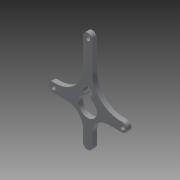
# Autodesk Inventor part: Fish Rib
Saved by Autodesk Inventor 2015 (Build 190159000, 159)
## iProperties
Created: 2014-11-02
Part Number: Fish Rib
Material: Generic
Document SubType Name: Modeling
Designer: Ryan
Density: 1 g/cm^3
Appearance: Default
Mass: 1.22571 g
Surface Area: 15.6256 cm^2
Volume: 1.22571 cm^3
Author: Ryan
Autodesk Inventor part; units mm, degrees
ref_plane "YZ Plane" through (0, 0, 0) normal (1, 0, 0) x (0, 1, 0)
ref_plane "XZ Plane" through (0, 0, 0) normal (0, 1, 0) x (-1, 0, 0)
ref_plane "XY Plane" through (0, 0, 0) normal (0, 0, 1) x (1, 0, 0)
sketch "Sketch1" plane through (0, 0, 0) normal (0, 0, 1) x (1, 0, 0)
  line L0 (0, 0) -> (0, 25.4)
  line L1 (0, 0) -> (0, -25.4)
  line L2 (-19.0266, -7.6091) -> (19.0734, -7.6091)
  circle A0 centre (0, 0) radius 2.54
  circle A1 centre (0, 25.4) radius 2.54
  circle A2 centre (-19.0266, -7.6091) radius 2.54
  circle A3 centre (19.0734, -7.6091) radius 2.54
  circle A4 centre (0, -25.4) radius 2.54
  circle A5 centre (0.0234, -7.6091) radius 5.08
  arc A6 (-1.9812, -2.9413) -> (-1.7729, -1.8189) centre (-2.2521, -2.3105) ccw
  arc A7 (1.7485, -1.8423) -> (1.9483, -2.9079) centre (2.1929, -2.3105) ccw
  line L3 (-2.54, 25.4) -> (-2.54, 10.1709)
  line L4 (2.54, 25.4) -> (2.54, 10.1709)
  line L5 (-2.54, -25.4) -> (-2.54, -19.0391)
  line L6 (2.54, -25.4) -> (2.54, -19.0391)
  line L7 (19.0734, -10.1491) -> (11.43, -10.1491)
  line L8 (19.0734, -5.0691) -> (17.78, -5.0691)
  line L9 (-19.0266, -5.0691) -> (-17.78, -5.0691)
  line L10 (-19.0266, -10.1491) -> (-11.43, -10.1491)
  arc A8 (-17.78, -5.0691) -> (-2.54, 10.1709) centre (-17.78, 10.1709) ccw
  arc A9 (2.54, 10.1709) -> (17.78, -5.0691) centre (17.78, 10.1709) ccw
  arc A10 (-2.54, -19.0391) -> (-11.43, -10.1491) centre (-11.43, -19.0391) ccw
  arc A11 (11.43, -10.1491) -> (2.54, -19.0391) centre (11.43, -19.0391) ccw
  circle A12 centre (-19.0266, -7.6091) radius 1.27
  circle A13 centre (0, 25.4) radius 1.27
  circle A14 centre (19.0734, -7.6091) radius 1.27
  dimension "d0" = 25.4
  dimension "d1" = 25.4
  dimension "d2" = 38.1
  dimension "d3" = 38.1
  dimension "d5" = 5.08
  dimension "d6" = 5.08
  dimension "d7" = 5.08
  dimension "d8" = 5.08
  dimension "d9" = 7.6091
  dimension "d10" = 5.08
  dimension "d12" = 4.445
  dimension "d13" = 35.56
  dimension "d14" = 22.86
  dimension "d15" = 10.16
  dimension "d16" = 2.54
  dimension "d17" = 2.54
  dimension "d18" = 2.54
  constraints: 24 point on circle, 23 end point, 20 tangent, 15 centre point, 8 coincident, 6 vertical, 5 horizontal, 3 horizontal alignment, 1 midpoint
  measures "d0" distance of L0.end L0.start
  measures "d1" distance of L0.start L1.end
  measures "d2" distance of L0.end L2.start
  measures "d3" distance of L2.start L2.end
  measures "d5" diameter of A4
  measures "d6" diameter of A3
  measures "d7" diameter of A2
  measures "d8" diameter of A1
  measures "d9" vertical distance of point (0.023, -7.609) L0.start
  measures "d10" diameter of A0
  measures "d12" distance of A6.centre A7.centre
  measures "d13" distance of A9.centre A8.centre
  measures "d14" distance of A11.centre A10.centre
  measures "d15" diameter of A5
  measures "d16" diameter of A13
  measures "d17" diameter of A14
  measures "d18" diameter of A12
extrude "Extrusion1" add sketch "Sketch1" along normal blind 2.54 contours A0 A6 A5 L2 A2 L9 A8 L3 A1 L0 | L0 A1 L4 A9 L8 A3 L2 A5 A7 A0 | A1 | A5 L1 A4 L5 A10 L10 A2 L2 | A5 L2 A3 L7 A11 L6 A4 L1 | A2 | A4 | A3
body "Solid1"
